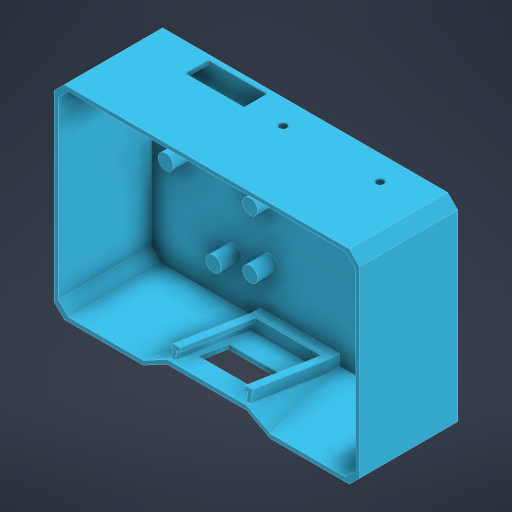
# Autodesk Inventor part: BasePlate
Saved by Autodesk Inventor 2024.2 (Build 282272000, 272)
## iProperties
Created: 2024-06-03
Part Number: BasePlate
Material: PBT Plastic
Document SubType Name: Modeling
Designer: simon
Density: 1.31 g/cm^3
Appearance: Turquoise
Author: simon
Autodesk Inventor part; units mm, degrees
ref_plane "YZ Plane" through (0, 0, 0) normal (1, 0, 0) x (0, 1, 0)
ref_plane "XZ Plane" through (0, 0, 0) normal (0, 1, 0) x (-1, 0, 0)
ref_plane "XY Plane" through (0, 0, 0) normal (0, 0, 1) x (1, 0, 0)
sketch "Sketch1" plane through (0, 0, 0) normal (0, 0, 1) x (1, 0, 0)
  line L0 (0, 0) -> (120, 0)
  line L1 (120, 0) -> (120, 80)
  line L2 (120, 80) -> (0, 80)
  line L3 (0, 80) -> (0, 0)
  dimension "d0" = 120
  dimension "d1" = 80
  constraints: 8 end point, 2 parallel, 1 horizontal, 1 perpendicular
  measures "d0" distance of L2.end L1.end
  measures "d1" distance of L1.end L0.end
extrude "Extrusion1" add sketch "Sketch1" along normal blind 2
sketch "Sketch2" plane through (0, 0, 2) normal (0, 0, 1) x (1, 0, 0)
  line L0 (0, 80) -> (0, 0) projected
  line L1 (120, 0) -> (120, 80) projected
  line L2 (0, 0) -> (120, 0)
  line L3 (120, 0) -> (120, 1.6)
  line L4 (120, 1.6) -> (0, 1.6)
  line L5 (0, 1.6) -> (0, 0)
  point P0 (0, 1.6)
  dimension "d4" = 1.6
  constraints: 8 end point, 2 parallel, 1 horizontal, 1 perpendicular, 1 point on line
  measures "d4" distance between parallel lines of L2 L4
extrude "Extrusion2" add sketch "Sketch2" along normal blind 5
ref_plane "Work Plane1" through (60, 0, 0) normal (1, 0, 0) x (0, 0, -1)
sketch "Sketch4" plane through (60, 0, 0) normal (1, 0, 0) x (0, 0, -1)
  line L0 (0, 0) -> (-7, 0) projected
  line L1 (-7, 0) -> (-38.6, 5)
  line L2 (-38.6, 5) -> (-38.6, 6.6)
  line L3 (-7, 1.6) -> (-7, 0) projected
  line L4 (-38.6, 6.6) -> (-7, 1.6)
  point P0 (-38.6, 5.8)
  dimension "d11" = 31.6
  dimension "d12" = 5
  constraints: 6 end point, 1 midpoint, 1 parallel, 1 perpendicular
  measures "d11" distance from line of point (-38.6, 5.8) L3
  measures "d12" distance from line of L1.end L0
extrude "Extrusion3" add sketch "Sketch4" along normal mid plane 31.2
sketch "Sketch5" plane through (44.4, 0, 7) normal (0, -0.9877122, 0.1562836) x (1, 0, 0)
  line L0 (3.6, 23.3931) -> (27.6, 23.3931)
  line L1 (27.6, 23.3931) -> (27.6, 11.3931)
  line L2 (27.6, 11.3931) -> (3.6, 11.3931)
  line L3 (3.6, 11.3931) -> (3.6, 23.3931)
  line L4 (0, 31.9931) -> (31.2, 31.9931) projected
  line L5 (0, 0) -> (0, 31.9931) projected
  point P0 (-44.4, -6.914)
  dimension "d15" = 24
  dimension "d16" = 12
  dimension "d17" = 8.6
  dimension "d18" = 3.6
  constraints: 8 end point, 2 parallel, 1 horizontal, 1 perpendicular
  measures "d15" distance of L1.end L2.end
  measures "d16" distance of L0.end L1.end
  measures "d17" distance between parallel lines of L4 L0
  measures "d18" distance between parallel lines of L5 L3
extrude "Extrusion4" cut sketch "Sketch5" against normal blind 2
sketch "Sketch6" plane through (44.4, 6.6, 38.6) normal (0, 0.9877122, -0.1562836) x (1, 0, 0)
  line L0 (31.2, 31.9931) -> (31.2, 0) projected
  line L1 (0, 0) -> (0, 31.9931) projected
  line L2 (31.2, 31.6441) -> (0, 31.6441)
  line L3 (0, 31.6441) -> (0, 33.2441)
  line L4 (0, 33.2441) -> (31.2, 33.2441)
  line L5 (31.2, 33.2441) -> (31.2, 31.6441)
  line L6 (3.6, 20.8501) -> (27.6, 20.8501) projected
  point P0 (-44.4, 39.1572)
  point P1 (0, 31.6441)
  dimension "d21" = 1.6
  dimension "d22" = 10.794
  constraints: 8 end point, 2 parallel, 2 point on line, 1 horizontal, 1 perpendicular
  measures "d21" distance between parallel lines of L4 L2
  measures "d22" distance between parallel lines of L6 L2
extrude "Extrusion5" add sketch "Sketch6" along normal blind 4.6
sketch "Sketch7" plane through (44.4, 1.6546, 7.3448) normal (0, 0.1562836, 0.9877122) x (1, 0, 0)
  line L0 (31.2, 0) -> (31.2, -1.5803) projected
  line L1 (0, 4.6) -> (31.2, 4.6) projected
  line L2 (31.2, 0) -> (29.6, 0)
  line L3 (29.6, 0) -> (29.6, 4.6)
  line L4 (29.6, 4.6) -> (31.2, 4.6)
  line L5 (31.2, 4.6) -> (31.2, 0)
  line L6 (0, 0) -> (-44.4, 0) projected
  line L7 (0, 0) -> (1.6, 0)
  line L8 (1.6, 0) -> (1.6, 4.6)
  line L9 (1.6, 4.6) -> (0, 4.6)
  line L10 (0, 4.6) -> (0, 0)
  line L11 (29.6, 4.6) -> (28.4, 4.6)
  line L12 (28.4, 4.6) -> (28.4, 3)
  line L13 (28.4, 3) -> (29.6, 3)
  line L14 (29.6, 3) -> (29.6, 4.6)
  line L15 (1.6, 4.6) -> (2.8, 4.6)
  line L16 (2.8, 4.6) -> (2.8, 3)
  line L17 (2.8, 3) -> (1.6, 3)
  line L18 (1.6, 3) -> (1.6, 4.6)
  point P0 (-44.4, -0.4864)
  point P1 (1.6, 3)
  point P2 (2.8, 4.6)
  dimension "d25" = 1.6
  dimension "d26" = 1.6
  dimension "d27" = 1.2
  dimension "d28" = 1.6
  dimension "d29" = 1.2
  dimension "d30" = 1.6
  constraints: 32 end point, 8 parallel, 4 horizontal, 4 perpendicular, 2 point on line
  measures "d25" distance between parallel lines of L5 L3
  measures "d26" distance between parallel lines of L10 L8
  measures "d27" distance of L13.end L12.end
  measures "d28" distance of L12.end L11.end
  measures "d29" distance of L16.end L17.end
  measures "d30" distance of L15.end L16.end
extrude "Extrusion6" add sketch "Sketch7" along normal blind 30
sketch "Sketch8" plane through (0, 0, 2) normal (0, 0, 1) x (1, 0, 0)
  line L0 (0, 1.6) -> (120, 1.6) projected
  line L1 (75.6, 1.6) -> (74, 1.6)
  line L2 (74, 1.6) -> (74, 5.93)
  line L3 (74, 5.93) -> (75.6, 5.93)
  line L4 (75.6, 5.93) -> (75.6, 1.6)
  line L5 (44.4, 1.6) -> (46, 1.6)
  line L6 (46, 1.6) -> (46, 5.93)
  line L7 (46, 5.93) -> (44.4, 5.93)
  line L8 (44.4, 5.93) -> (44.4, 1.6)
  line L9 (0, 80) -> (0, 1.6) projected
  line L10 (75.6, 5.93) -> (44.4, 5.93)
  line L11 (44.4, 5.93) -> (44.4, 4.33)
  line L12 (44.4, 4.33) -> (75.6, 4.33)
  line L13 (75.6, 4.33) -> (75.6, 5.93)
  point P0 (0, 0)
  point P1 (74.8, 5.93)
  point P2 (74, 4.33)
  point P3 (46, 4.33)
  dimension "d33" = 1.6
  dimension "d34" = 4.33
  dimension "d35" = 1.6
  dimension "d36" = 4.33
  dimension "d37" = 28
  dimension "d38" = 44.4
  dimension "d39" = 1.6
  constraints: 24 end point, 6 parallel, 3 horizontal, 3 perpendicular, 3 point on line, 1 midpoint
  measures "d33" distance of L2.end L3.end
  measures "d34" distance from line of point (74.8, 5.93) L0
  measures "d35" distance of L7.end L6.end
  measures "d36" distance of L6.end L5.end
  measures "d37" distance between parallel lines of L6 L2
  measures "d38" distance between parallel lines of L9 L8
  measures "d39" distance between parallel lines of L12 L10
extrude "Extrusion7" add sketch "Sketch8" along normal blind 4 contours L8 L12 L6 L0 | L8 L7 L6 L12 | L2 L12 L4 L0 | L6 L10 L2 L12 | L2 L3 L4 L12
sketch "Sketch10" plane through (0, 0, 7) normal (0, 0, 1) x (1, 0, 0)
  line L0 (0, 0) -> (44.4, 0) projected
  line L1 (0, 1.6) -> (120, 1.6) projected
  line L2 (0, 0) -> (35, 0)
  line L3 (35, 0) -> (35, 1.6)
  line L4 (35, 1.6) -> (0, 1.6)
  line L5 (0, 1.6) -> (0, 0)
  line L6 (120, 0) -> (120, 80) projected
  line L7 (0, 0) -> (120, 0) projected
  line L8 (120, 1.6) -> (85, 1.6)
  line L9 (85, 1.6) -> (85, 0)
  line L10 (85, 0) -> (120, 0)
  line L11 (120, 0) -> (120, 1.6)
  point P0 (44.4, 1.6)
  point P1 (0, 0.8)
  point P2 (35, 0.8)
  point P3 (120, 0.8)
  point P4 (85, 0.8)
  dimension "d42" = 35
  dimension "d43" = 35
  constraints: 16 end point, 4 midpoint, 4 parallel, 4 point on line, 2 horizontal, 2 perpendicular
  measures "d42" distance of point (0, 0.8) point (35, 0.8)
  measures "d43" distance of point (120, 0.8) point (85, 0.8)
extrude "Extrusion8" add sketch "Sketch10" along normal blind 31.6 contours L5 L1 L3 L0 | L9 L1 L6 L7
ref_plane "Work Plane8" through (35, 0, 38.6) normal (0.4650968, -0.874382, 0.1383516) x (0.2851209, 0, -0.9584916)
sketch "Sketch12" plane through (35, 0, 38.6) normal (0.4650968, -0.874382, 0.1383516) x (0.2851209, 0, -0.9584916)
  line L0 (30.2883, -7.878) -> (32.9685, 0) projected
  line L1 (30.2883, -7.878) -> (0, 0) projected
  line L2 (32.9685, 0) -> (0, 0)
  line L3 (2.6801, 10.3042) -> (11.5759, 36.4526) projected
  line L4 (0, 0) -> (2.6801, 10.3042)
  line L5 (2.6801, 10.3042) -> (32.9685, 0)
  point P0 (27.0185, -38.9562)
  constraints: 6 end point, 1 horizontal, 1 perpendicular
ref_plane "Work Plane9" through (75.6, 0, 7) normal (0.4650968, 0.874382, -0.1383516) x (0, 0.1562836, 0.9877122)
sketch "Sketch13" plane through (75.6, 0, 7) normal (0.4650968, 0.874382, -0.1383516) x (0, 0.1562836, 0.9877122)
  line L0 (31.9931, 0) -> (0, 0) projected
  line L1 (31.4618, 9.8833) -> (31.2117, 10.6184) projected
  line L2 (0, 0) -> (31.2117, 10.6184)
  line L3 (32.2432, -0.735) -> (31.9931, 0) projected
  line L4 (31.2117, 10.6184) -> (31.9931, 0)
  line L5 (31.9931, 0) -> (0, 0)
  point P0 (-6.914, -67.4345)
  constraints: 6 end point, 1 horizontal, 1 perpendicular
sketch3d "3D Sketch1"
  line L0 (44.4, 5, 38.6) -> (44.4, 6.6, 38.6)
sweep "Sweep1" add profiles "Sketch12" path "3D Sketch1" contours L2 L4 L5
sketch3d "3D Sketch2"
  line L0 (75.6, 5, 38.6) -> (75.6, 6.6, 38.6)
sweep "Sweep2" add profiles "Sketch13" path "3D Sketch2"
ref_plane "Work Plane13" through (44.4, 0, 7) normal (0, -1, 0) x (-0.2851209, 0, 0.9584916)
sketch "Sketch22" plane through (44.4, 0, 7) normal (0, -1, 0) x (-0.2851209, 0, 0.9584916)
  line L0 (0, 0) -> (-4.7925, 1.4256) projected
  line L1 (0, 0) -> (2.6801, 9.0098)
  line L2 (2.6801, 9.0098) -> (32.9685, 0)
  line L3 (32.9685, 0) -> (0, 0)
  point P0 (5.9499, 44.5529)
  point P1 (-14.3774, 4.2768)
  constraints: 6 end point, 1 horizontal, 1 perpendicular
sketch3d "3D Sketch3"
  line L0 (35, 0, 38.6) -> (35, 1.6, 38.6)
sweep "Sweep3" add profiles "Sketch22" path "3D Sketch3"
ref_plane "Work Plane14" through (75.6, 0, 7) normal (0, -1, 0) x (1, 0, 0)
sketch "Sketch23" plane through (75.6, 0, 7) normal (0, -1, 0) x (1, 0, 0)
  line L0 (0, 0) -> (9.4, 0) projected
  line L1 (9.4, 0) -> (0, 0)
  line L2 (0, 31.6) -> (9.4, 31.6) projected
  line L3 (0, 0) -> (9.4, 31.6)
  line L4 (9.4, 31.6) -> (9.4, 0)
  point P0 (-75.6, -7)
  constraints: 6 end point, 1 collinear, 1 perpendicular
sketch3d "3D Sketch4"
  line L0 (85, 0, 38.6) -> (85, 1.6, 38.6)
sweep "Sweep4" add profiles "Sketch23" path "3D Sketch4"
sketch "Sketch24" plane through (0, 0, 2) normal (0, 0, 1) x (1, 0, 0)
  line L0 (120, 80) -> (0, 80) projected
  line L1 (0, 0) -> (1.6, 0)
  line L2 (1.6, 0) -> (1.6, 80)
  line L3 (1.6, 80) -> (0, 80)
  line L4 (0, 80) -> (0, 0)
  line L5 (120, 1.6) -> (120, 80) projected
  line L6 (0, 80) -> (120, 80)
  line L7 (120, 80) -> (120, 78.4)
  line L8 (120, 78.4) -> (0, 78.4)
  line L9 (0, 78.4) -> (0, 80)
  line L10 (120, 80) -> (118.4, 80)
  line L11 (118.4, 80) -> (118.4, 0)
  line L12 (118.4, 0) -> (120, 0)
  line L13 (120, 0) -> (120, 80)
  point P0 (1.6, 78.4)
  point P1 (118.4, 78.4)
  dimension "d61" = 1.6
  dimension "d62" = 1.6
  dimension "d63" = 1.6
  constraints: 24 end point, 6 parallel, 3 horizontal, 3 perpendicular, 3 point on line
  measures "d61" distance of L3.end L2.end
  measures "d62" distance of L6.end L7.end
  measures "d63" distance of L12.end L11.end
extrude "Extrusion11" add sketch "Sketch24" along normal blind 36.6
chamfer "Chamfer1" distance 4 angle 45 8 edges at (0, 0, 19.3) (0, 80, 19.3) (120, 0, 19.3) (120, 80, 19.3) (118.4, 78.4, 20.3) (1.6, 78.4, 20.3) (118.4, 1.6, 20.3) (1.6, 1.6, 20.3)
sketch "Sketch25" plane through (4, 80, 0) normal (0, 1, 0) x (1, 0, 0)
  line L0 (110.4, -2) -> (1.6, -2) projected
  line L1 (20, -2) -> (43, -2)
  line L2 (43, -2) -> (43, -11)
  line L3 (43, -11) -> (20, -11)
  line L4 (20, -11) -> (20, -2)
  line L5 (-4, 0) -> (-4, -38.6) projected
  dimension "d69" = 23
  dimension "d70" = 9
  dimension "d71" = 24
  constraints: 8 end point, 2 parallel, 1 horizontal, 1 perpendicular, 1 point on line
  measures "d69" distance of L2.end L3.end
  measures "d70" distance of L1.end L2.end
  measures "d71" distance between parallel lines of L5 L4
extrude "Extrusion12" cut sketch "Sketch25" against normal blind 2
sketch "Sketch26" plane through (0, 0, 2) normal (0, 0, 1) x (1, 0, 0)
  line L0 (30.8, 69.4) -> (32.4, 69.4)
  line L1 (32.4, 69.4) -> (32.4, 63.4)
  line L2 (32.4, 63.4) -> (30.8, 63.4)
  line L3 (30.8, 63.4) -> (30.8, 69.4)
  line L4 (38.6, 69.4) -> (40.2, 69.4)
  line L5 (40.2, 69.4) -> (40.2, 63.4)
  line L6 (40.2, 63.4) -> (38.6, 63.4)
  line L7 (38.6, 63.4) -> (38.6, 69.4)
  line L8 (24, 80) -> (47, 80) projected
  line L9 (24, 80) -> (24, 78.4) projected
  point P0 (0, 0)
  dimension "d74" = 6
  dimension "d75" = 10.6
  dimension "d76" = 1.6
  dimension "d77" = 1.6
  dimension "d78" = 6.2
  dimension "d79" = 6.8
  constraints: 16 end point, 4 parallel, 2 horizontal, 2 perpendicular, 2 point on line
  measures "d74" distance of L2.end L0.start
  measures "d75" distance between parallel lines of L8 L0
  measures "d76" distance of L0.start L0.end
  measures "d77" distance of L4.start L4.end
  measures "d78" distance between parallel lines of L7 L1
  measures "d79" distance between parallel lines of L3 L9
extrude "Extrusion13" add sketch "Sketch26" along normal blind 9
sketch "Sketch27" plane through (4, 80, 0) normal (0, 1, 0) x (1, 0, 0)
  circle A0 centre (95.15, -9.7) radius 1.5
  circle A1 centre (57.05, -9.7) radius 1.5
  line L0 (116, -38.6) -> (116, 0) projected
  line L1 (112, 0) -> (0, 0) projected
  point P0 (-4, 0)
  dimension "d82" = 3
  dimension "d83" = 3
  dimension "d84" = 20.85
  dimension "d85" = 38.1
  dimension "d86" = 9.7
  dimension "d87" = 9.7
  constraints: 2 centre point
  measures "d82" diameter of A0
  measures "d83" diameter of A1
  measures "d84" distance from line of L0 A0.centre
  measures "d85" distance of A1.centre A0.centre
  measures "d86" distance from line of A0.centre L1
  measures "d87" distance from line of A1.centre L1
extrude "Extrusion14" cut sketch "Sketch27" against normal blind 2
sketch "Sketch28" plane through (0, 0, 2) normal (0, 0, 1) x (1, 0, 0)
  circle A0 centre (106.4, 46.4) radius 3
  circle A1 centre (106.4, 23.4) radius 3
  circle A2 centre (48.4, 46.4) radius 3
  circle A3 centre (48.4, 23.4) radius 3
  line L0 (118.4, 74.4) -> (118.4, 5.6) projected
  line L1 (5.6, 78.4) -> (114.4, 78.4) projected
  circle A4 centre (15.18, 45.05) radius 3
  circle A5 centre (33.96, 19.65) radius 3
  line L2 (1.6, 5.6) -> (1.6, 74.4) projected
  point P0 (0, 0)
  dimension "d90" = 6
  dimension "d91" = 6
  dimension "d92" = 6
  dimension "d93" = 6
  dimension "d94" = 23
  dimension "d95" = 23
  dimension "d96" = 58
  dimension "d97" = 12
  dimension "d98" = 32
  dimension "d101" = 6
  dimension "d102" = 6
  dimension "d103" = 33.35
  dimension "d104" = 13.58
  dimension "d105" = 32.36
  dimension "d106" = 58.75
  constraints: 6 centre point
  measures "d90" diameter of A0
  measures "d91" diameter of A1
  measures "d92" diameter of A2
  measures "d93" diameter of A3
  measures "d94" distance of A0.centre A1.centre
  measures "d95" distance of A2.centre A3.centre
  measures "d96" distance of A1.centre A3.centre
  measures "d97" distance from line of A1.centre L0
  measures "d98" distance from line of L1 A0.centre
  measures "d101" diameter of A4
  measures "d102" diameter of A5
  measures "d103" distance from line of L1 A4.centre
  measures "d104" distance from line of L2 A4.centre
  measures "d105" distance from line of L2 A5.centre
  measures "d106" distance from line of L1 A5.centre
extrude "Extrusion15" add sketch "Sketch28" along normal blind 8
body "Solid1"
